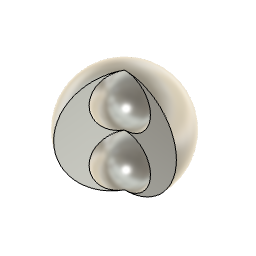
The2BallsHolder (Autodesk Fusion 360 design; units mm, degrees)
Autodesk Fusion 360 part; units mm, degrees
note: some values were not read from the file. Set by a fixed rule: which sketch regions a step uses.
sketch "Sketch1" plane through (0, 0, 0) normal (0, 1, 0) x (1, 0, 0)
  circle A0 centre (0, 0) radius 38.1
  line L0 (-38.1, 0) -> (44.45, 0)
  circle A1 centre (0, -19.05) radius 19.05
  circle A2 centre (0, 19.05) radius 19.05
  constraint coincident A0.centre origin
  constraint coincident A0 L0.start
  constraint horizontal L0
  constraint coincident A0.centre A1
  constraint tangent L0 A1
  constraint coincident A0.centre A2
  constraint tangent A1 A2
revolve "Revolve1" add sketch "Sketch1" angle 240 about axis through (0, 0, 1.75) along (0, 0, 1) contours A0 L0 A2 | A0 L0 A1 picked at (30.6127, 4.7243) picked at (30.6127, -4.7243)
